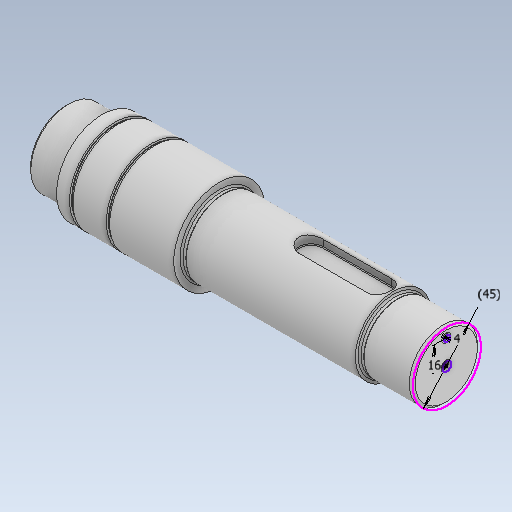
# Autodesk Inventor part: Тихоходный валл
Saved by Autodesk Inventor 2021 (Build 250183000, 183)
## iProperties
Created: 2023-05-07
Part Number: Тихоходный валл
Material: Типовые
Document SubType Name: Modeling
Designer: gdevc
Density: 1 g/cm^3
Appearance: По умолчанию
Mass: 538.484 g
Surface Area: 485.516 cm^2
Volume: 538.484 cm^3
Author: gdevc
Autodesk Inventor part; units mm, degrees
ref_plane "YZ Plane" through (0, 0, 0) normal (1, 0, 0) x (0, 1, 0)
ref_plane "XY Plane" through (0, 0, 0) normal (0, 0, 1) x (1, 0, 0)
sketch "Эскиз1" plane through (0, 0, 0) normal (0, 0, 1) x (1, 0, 0)
  line L0 (0, 0) -> (0, 25)
  line L1 (24, 25) -> (24, 30)
  line L2 (32.575, 30) -> (32.575, 28.5)
  line L3 (32.575, 28.5) -> (34.775, 28.5)
  line L4 (34.775, 28.5) -> (34.775, 30)
  line L5 (94.5, 30) -> (101.25, 30)
  line L6 (101.25, 30) -> (101.25, 25)
  line L7 (215.8, 25) -> (215.8, 22.5)
  line L8 (250.8, 22.5) -> (250.8, 0)
  line L9 (250.8, 0) -> (0, 0)
  line L10 (101.25, 25) -> (101.25, 24.875)
  line L11 (101.25, 24.875) -> (104.25, 24.875)
  line L12 (104.25, 24.875) -> (104.375, 25)
  line L13 (104.375, 25) -> (215.8, 25)
  line L14 (24, 25) -> (24, 24.75)
  line L15 (24, 24.75) -> (21, 24.75)
  line L16 (20.75, 25) -> (0, 25)
  line L17 (20.75, 25) -> (21, 24.75)
  line L18 (215.8, 22.5) -> (215.8, 22.25)
  line L19 (215.8, 22.25) -> (218.8, 22.25)
  line L20 (218.8, 22.25) -> (219.05, 22.5)
  line L21 (219.05, 22.5) -> (250.8, 22.5)
  line L22 (24, 30) -> (32.575, 30)
  line L23 (34.775, 30) -> (35.7524, 30)
  line L24 (35.7524, 30) -> (56.775, 30)
  line L25 (60.3, 30) -> (92.3, 30)
  line L26 (56.775, 30) -> (56.775, 28.5)
  line L27 (56.775, 28.5) -> (58.975, 28.5)
  line L28 (58.975, 28.5) -> (58.975, 30)
  line L29 (58.975, 30) -> (60.3, 30)
  line L30 (92.3, 30) -> (94.8795, 30)
  point P0 (92.3, 28.5)
  point P1 (94.5, 28.5)
  dimension "d4" = 24
  dimension "d6" = 2.2
  dimension "d7" = 57
  dimension "d12" = 35
  dimension "d13" = 250.8
  dimension "d49" = 45
  dimension "d50" = 3
  dimension "d51" = 50
  dimension "d52" = 49.75
  dimension "d55" = 50
  dimension "d56" = 0.25
  dimension "d57" = 45
  dimension "d58" = 3
  dimension "d61" = 45
  dimension "d62" = 45
  dimension "d63" = 0.25
  dimension "d64" = 3
  dimension "d67" = 10.775
  dimension "d70" = 77.25
  dimension "d72" = 60
  dimension "d73" = 60
  dimension "d74" = 60
  dimension "d76" = 2.2
  dimension "d77" = 57
  dimension "d78" = 22
  constraints: 62 end point, 9 perpendicular, 5 point on line, 5 vertical, 2 horizontal, 2 parallel
  measures "d4" distance from line of L0.start L1
  measures "d6" distance of L2.end L3.end
  measures "d7" diameter of L3 L9
  measures "d12" distance between parallel lines of L8 L7
  measures "d13" distance between parallel lines of L8 L0
  measures "d49" angle of L13 L12
  measures "d50" distance of L10.end L11.end
  measures "d51" diameter of L13 L9
  measures "d52" diameter of L11 L9
  measures "d55" diameter of L16 L9
  measures "d56" distance between parallel lines of L16 L15
  measures "d57" angle of L16 L17
  measures "d58" distance of L14.end L15.end
  measures "d61" diameter of L21 L9
  measures "d62" angle of L21 L20
  measures "d63" distance between parallel lines of L21 L19
  measures "d64" distance of L18.end L19.end
  measures "d67" distance between parallel lines of L1 L4
  measures "d70" distance between parallel lines of L6 L1
  measures "d72" diameter of L24 L9
  measures "d73" diameter of L22 L9
  measures "d74" diameter of L5 L9
  measures "d76" distance of L26.end L27.end
  measures "d77" diameter of L27 L9
  measures "d78" distance between parallel lines of L4 L26
revolve "Вращение1" add sketch "Эскиз1" angle 360 about axis through (250.8, 0, 0) along (-1, 0, 0)
fillet "Сопряжение1" radius 0.2 2 edges at (32.575, -28.5, 0) (34.775, -28.5, 0)
ref_plane "РабПлоскость1" through (0, 19, 0) normal (0, 1, 0) x (-1, 0, 0)
sketch "Эскиз2" plane through (0, 19, 0) normal (0, 1, 0) x (-1, 0, 0)
  line L0 (-161.7, -8) -> (-206.7, -8)
  line L1 (-206.7, -8) -> (-206.7, 8)
  line L2 (-206.7, 8) -> (-161.7, 8)
  line L3 (-161.7, 8) -> (-161.7, -8)
  line L4 (-103.5, 25) -> (-103.5, -25) projected
  arc A0 (-161.7, -8) -> (-161.7, 8) centre (-161.7, 0) ccw
  arc A1 (-206.7, 8) -> (-206.7, -8) centre (-206.7, 0) ccw
  point P0 (0, 0)
  dimension "d17" = 45
  dimension "d18" = 16
  dimension "d19" = 8
  dimension "d20" = 58.2
  constraints: 8 end point, 4 point on circle, 2 centre point, 2 midpoint, 2 parallel, 1 horizontal, 1 perpendicular, 1 point on line
  measures "d17" distance between parallel lines of L1 L3
  measures "d18" distance between parallel lines of L2 L0
  measures "d19" distance from line of point (0, 0) L0
  measures "d20" distance between parallel lines of L4 L3
extrude "Выдавливание1" cut sketch "Эскиз2" along normal blind 65.75
chamfer "Фаска1" distance 2 angle 45 2 edges at (250.8, -22.5, 0) (0, -25, 0)
fillet "Сопряжение3" radius 1 1 edges at (215.8, -22.25, 0)
fillet "Сопряжение3" radius 0.5 1 edges at (218.8, -22.25, 0)
sketch "Эскиз3" plane through (250.8, 0, 0) normal (1, 0, 0) x (0, 0, -1)
  circle A0 centre (0, 0) radius 22.5 projected
  circle A1 centre (0, 16) radius 2
  circle A2 centre (0, 0) radius 2.9879
  dimension "d28" = 45
  dimension "d29" = 16
  dimension "d30" = 4
  constraints: 2 centre point, 1 coincident
  measures "d28" diameter of A0
  measures "d29" distance of point (0, 0) A1.centre
  measures "d30" diameter of A1
hole "Отверстие1" at (250.8, 16, 0) direction (-1, 0, 0) diameter 4 depth 12 tip angle 118
hole "Отверстие2" at (250.8, 0, 0) direction (-1, 0, 0) diameter 4.917 depth 18 tip angle 118 thread size "M6x1" class "6H" standard "ISO Metric profile"
chamfer "Фаска2" distance 1 angle 45 2 edges at (250.8, 0, 2.4585) (250.8, 16, 2)
fillet "Сопряжение4" radius 0.5 4 edges at (184.2, 19, 8) (214.7, 19, 0) (184.2, 19, -8) (153.7, 19, 0)
fillet "Сопряжение5" radius 1 1 edges at (101.25, -24.875, 0)
fillet "Сопряжение6" radius 0.5 1 edges at (104.25, -24.875, 0)
fillet "Сопряжение7" radius 0.5 1 edges at (21, -24.75, 0)
fillet "Сопряжение7" radius 1 1 edges at (24, -24.75, 0)
fillet "Сопряжение8" [suppressed]
fillet "Сопряжение9" radius 0.2 2 edges at (56.775, -28.5, 0) (58.975, -28.5, 0)
equation "\"d19\" = 0.5 * d18"
